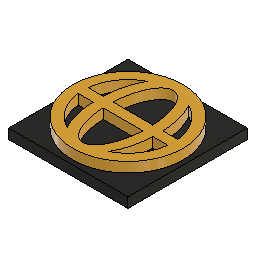
icon_www (Autodesk Fusion 360 design; units mm, degrees)
Autodesk Fusion 360 part; units mm, degrees
sketch "Sketch1" plane through (0, 0, 0) normal (0, 0, 1) x (1, 0, 0)
  line L0 (5.95, -5.95) -> (-5.95, -5.95)
  line L1 (-5.95, -5.95) -> (-5.95, 5.95)
  line L2 (-5.95, 5.95) -> (5.95, 5.95)
  line L3 (5.95, 5.95) -> (5.95, -5.95)
  line L4 (5.95, -5.95) -> (-5.95, 5.95) construction
  line L5 (-5.95, -5.95) -> (5.95, 5.95) construction
  circle A0 centre (0, 0) radius 5.5
  arc A1 (-2.058, 4.0018) -> (-4.4755, 0.4687) centre (0, 0) ccw
  arc A2 (-4.4755, -0.4687) -> (-2.058, -4.0018) centre (0, 0) ccw
  ellipse E0 centre (0, 0) end of major axis (3, 0) minor radius 5.5 (-2.058, 4.0018) -> (-2.9876, 0.5) ccw
  ellipse E1 centre (0, 0) end of major axis (3, 0) minor radius 5.5 (-2.9876, -0.5) -> (-2.058, -4.0018) ccw
  arc A3 (2.058, -4.0018) -> (4.4721, -0.5) centre (0, 0) ccw
  arc A4 (4.4721, 0.5) -> (2.058, 4.0018) centre (0, 0) ccw
  line L6 (2.9876, 0.5) -> (4.4721, 0.5)
  ellipse E2 centre (0, 0) end of major axis (3, 0) minor radius 5.5 (2.058, -4.0018) -> (2.9876, -0.5) ccw
  ellipse E3 centre (0, 0) end of major axis (3, 0) minor radius 5.5 (2.9876, 0.5) -> (2.058, 4.0018) ccw
  ellipse E4 centre (0, 0) end of major axis (2, 0) minor radius 4.5 (-1.9876, -0.5) -> (1.9876, -0.5) ccw
  ellipse E5 centre (0, 0) end of major axis (2, 0) minor radius 4.5 (1.9876, 0.5) -> (-1.9876, 0.5) ccw
  line L7 (4.4721, -0.5) -> (2.9876, -0.5)
  line L8 (1.9876, -0.5) -> (-1.9876, -0.5)
  line L9 (-2.9876, -0.5) -> (-4.4721, -0.5)
  line L10 (-4.4721, 0.5) -> (-2.9876, 0.5)
  line L11 (-1.9876, 0.5) -> (1.9876, 0.5)
  dimension "d1" = 11.9
  dimension "d2" = 11.9
  constraint horizontal L0
  constraint perpendicular L0 L1
  constraint parallel L0 L2
  constraint parallel L1 L3
  constraint concentric A0 A1
  constraint concentric A0 E0
  constraint concentric A1 A3
  constraint coincident A3.start E0
  constraint concentric E0 E2
  constraint horizontal L7
  constraint parallel L7 L10
  constraint coincident A0.centre A1.centre
  constraint coincident L10.start A1
  constraint coincident L9.end A1
  constraint coincident A2.start A1
  constraint concentric A1 A2
  constraint concentric E0 E1
  constraint coincident L11.start L10
  constraint coincident L8.end L7
  constraint coincident L9.start L7
  constraint coincident A4.start A3
  constraint concentric A3 A4
  constraint coincident L11.end E4
  constraint coincident L6.start E2
  constraint collinear L6 L10
  constraint concentric E2 E3
  constraint coincident L8.start L7
  constraint concentric E4 E5
  constraint collinear L7 L8
  constraint collinear L8 L9
  constraint collinear L10 L11
  measures "d1" distance of L1.end L2.end
  measures "d2" distance of L0.end L1.end
extrude "Extrude1" add sketch "Sketch1" against normal blind 1 contours L0 L1 L2 L3 | A0 | A1 E0 L10 | A2 E1 L9 | A3 E2 L7 | A4 L6 E3 | E4 L8 | E5 L11
extrude "Extrude3" add sketch "Sketch1" along normal blind 1 contours A0
